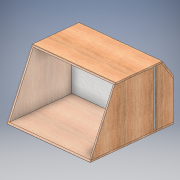
# Autodesk Inventor part: spraybooth
Saved by Autodesk Inventor 2017 (Build 210142000, 142)
## iProperties
Created: 2019-04-06
Part Number: spraybooth
Material: Wood (Birch)
Document SubType Name: Modeling
Designer: Brian
Density: 0.55 g/cm^3
Appearance: Birch - Natural Polished
plywood_thickness: 0.500 in
full_depth: 26.000 in
filter_width: 25.000 in
twobyfour_height: 3.500 in
filter_thickness: 1.000 in
acrylic_thickness: 0.250 in
filter_height: 16.000 in
front_angle: 65.00 deg
plenum_depth: 4.250 in
twobyfour_thickness: 1.500 in
d42: 0.500 in
d86: 25.500 in
d87: 0.00 deg
d90: 1.000 in
d93: 0.500 in
d96: 0.500 in
d102: 0.500 in
d104: 1.000 in
d105: 3.500 in
d106: 1.000 in
d109: 25.000 in
d110: 0.00 deg
d111: 25.000 in
d112: 0.00 deg
d113: 1.500 in
d114: 0.00 deg
d115: 1.500 in
d116: 0.00 deg
d117: 1.000 in
d118: 0.00 deg
d123: 25.500 in
d124: 0.00 deg
d129: 1.000 in
d130: 0.00 deg
d131: 25.000 in
d132: 0.00 deg
d133: 25.000 in
d134: 0.00 deg
d137: 0.500 in
d138: 0.00 deg
d139: 25.500 in
d140: 0.00 deg
d143: 0.00 deg
d144: 1.500 in
d145: 0.00 deg
d146: 0.500 in
d147: 0.00 deg
d148: 25.500 in
d149: 0.00 deg
d150: 0.500 in
d151: 0.00 deg
d152: 0.500 in
d153: 0.00 deg
d154: 0.500 in
d155: 0.00 deg
d156: 0.500 in
d157: 0.00 deg
d158: 0.500 in
d159: 0.00 deg
d160: 0.500 in
d161: 0.00 deg
d59: 6.070 in
d61: 14.020 in
d62: 11.582 in
d63: 18.641 in
d65: 19.517 in
d66: 35.88 deg
d120: 12.056 in
Author: Brian
Autodesk Inventor part; units mm, degrees
ref_plane "YZ Plane" through (0, 0, 0) normal (1, 0, 0) x (0, 1, 0)
ref_plane "XZ Plane" through (0, 0, 0) normal (0, 1, 0) x (-1, 0, 0)
ref_plane "XY Plane" through (0, 0, 0) normal (0, 0, 1) x (1, 0, 0)
sketch "Sketch2" plane through (0, 0, 0) normal (1, 0, 0) x (0, 0, 1)
  line L0 (-641.7779, 0) -> (-641.7779, -290.0603)
  line L1 (-654.4779, -294.1723) -> (-654.4779, 0)
  line L2 (-551.5263, -419.1) -> (-195.4295, -419.1)
  line L3 (5.9221, 12.7) -> (-654.4779, 12.7)
  line L4 (-654.4779, 12.7) -> (-654.4779, 0)
  line L5 (11.6772, 10.0164) -> (5.9221, 12.7)
  line L6 (0, 0) -> (5.9221, 12.7)
  line L7 (-573.2932, -406.4) -> (-654.4779, -294.1723)
  line L8 (-521.1279, -406.4) -> (-533.8279, -406.4)
  line L9 (-533.8279, 0) -> (-521.1279, 0)
  line L10 (-559.2279, -317.5) -> (-533.8279, -317.5)
  line L11 (-533.8279, 0) -> (-559.2279, 0)
  line L12 (-641.7779, -88.9) -> (-533.8279, -88.9)
  line L13 (-521.1279, -406.4) -> (-533.8279, -406.4)
  line L14 (-533.8279, -406.4) -> (-533.8279, -381)
  line L15 (-521.1279, -381) -> (-521.1279, -406.4)
  line L16 (-521.1279, 0) -> (-533.8279, 0)
  line L17 (-533.8279, 0) -> (-533.8279, -25.4)
  line L18 (-533.8279, -25.4) -> (-521.1279, -25.4)
  line L19 (-521.1279, -25.4) -> (-521.1279, 0)
  line L20 (-495.7279, 0) -> (-521.1279, 0)
  line L21 (-551.5263, -419.1) -> (-564.1061, -419.1)
  line L22 (5.9221, 12.7) -> (11.6772, 10.0164)
  line L23 (11.6772, 10.0164) -> (-188.4231, -419.1)
  line L24 (-188.4231, -419.1) -> (-194.1781, -416.4164)
  line L25 (-654.4779, 0) -> (-641.7779, 0)
  line L26 (-641.7779, 0) -> (-654.4779, 0)
  line L27 (-641.7779, 0) -> (-654.4779, 0)
  line L28 (-521.1279, -25.4) -> (-533.8279, -25.4)
  line L29 (-533.8279, 0) -> (-521.1279, 0)
  line L30 (-521.1279, -406.4) -> (-533.8279, -406.4)
  line L31 (-559.2279, -317.5) -> (-533.8279, -317.5)
  line L32 (-533.8279, -88.9) -> (-641.7779, -88.9)
  line L33 (-521.1279, -381) -> (-521.1279, -25.4)
  line L34 (5.9221, 12.7) -> (11.6772, 10.0164)
  line L35 (-521.1279, -406.4) -> (-533.8279, -406.4)
  line L36 (-533.8279, -406.4) -> (-533.8279, -381)
  line L37 (-521.1279, -381) -> (-521.1279, -406.4)
  line L38 (-533.8279, -25.4) -> (-521.1279, -25.4)
  line L39 (-521.1279, -25.4) -> (-521.1279, -381)
  line L40 (-521.1279, -25.4) -> (-533.8279, -25.4)
  line L41 (-533.8279, -25.4) -> (-533.8279, 0)
  line L42 (-533.8279, 0) -> (-521.1279, 0)
  line L43 (-521.1279, 0) -> (-521.1279, -25.4)
  line L44 (-654.4779, -294.1723) -> (-573.2932, -406.4)
  line L45 (-564.1061, -419.1) -> (-551.5263, -419.1)
  line L46 (-533.8279, -406.4) -> (-557.6186, -406.4)
  line L47 (-495.7279, -406.4) -> (-521.1279, -406.4)
  line L48 (-194.1781, -416.4164) -> (0, 0)
  line L49 (-521.1279, -381) -> (-533.8279, -381)
  line L50 (-557.6186, -406.4) -> (-573.2932, -406.4)
  line L51 (-521.1279, -406.4) -> (-495.7279, -406.4)
  line L52 (-495.7279, -406.4) -> (-495.7279, 0)
  line L53 (-189.5074, -406.4) -> (-495.7279, -406.4)
  line L54 (0, 0) -> (-495.7279, 0)
  line L55 (-559.2279, 0) -> (-641.7779, 0)
  line L56 (-533.8279, -25.4) -> (-533.8279, -88.9)
  line L57 (-533.8279, -88.9) -> (-533.8279, -317.5)
  line L58 (-533.8279, -381) -> (-533.8279, -317.5)
  line L59 (-559.2279, -317.5) -> (-621.9282, -317.5)
  line L60 (-557.6186, -406.4) -> (-621.9282, -317.5)
  line L61 (-573.2932, -406.4) -> (-564.1061, -419.1)
  line L62 (-621.9282, -317.5) -> (-654.4779, -272.5041)
  line L63 (-189.5074, -406.4) -> (-189.5074, -406.4)
  line L64 (-189.5074, -406.4) -> (-194.1781, -416.4164)
  line L65 (-195.4295, -419.1) -> (-189.5074, -406.4)
  point P0 (-641.7779, -285.2823)
  dimension "d42" = 12.7
  dimension "full_depth" = 660.4
  dimension "d59" = 154.1882
  dimension "d61" = 356.0967
  dimension "d62" = 294.1723
  dimension "d63" = 473.4775
  dimension "d65" = 495.7279
  dimension "d66" = 35.882
  dimension "d90" = 25.4
  dimension "twobyfour_height" = 88.9
  dimension "d93" = 12.7
  dimension "filter_thickness" = 25.4
  dimension "d96" = 12.7
  dimension "acrylic_thickness" = 6.35
  dimension "d102" = 12.7
  dimension "filter_height" = 406.4
  dimension "d104" = 25.4
  dimension "d105" = 88.9
  dimension "d106" = 25.4
  dimension "front_angle" = 65
  dimension "d120" = 306.2205
  dimension "plenum_depth" = 107.95
  constraints: 135 end point, 15 collinear, 14 horizontal, 13 parallel, 11 perpendicular, 6 point on line, 1 vertical
  measures "d42" distance between parallel lines of L1 L0
  measures "full_depth" distance of L3.start L4.start
  measures "d59" distance of L21.end L1.start
  measures "d61" distance of L2.end L2.start
  measures "d62" distance of L1.end L1.start
  measures "d63" distance of L23.end L5.start
  measures "d65" distance of L6.start L20.start
  measures "d66" angle of L1 L7
  measures "d90" distance between parallel lines of L49 L8
  measures "twobyfour_height" distance between parallel lines of L10 L46
  measures "d93" distance between parallel lines of L2 L53
  measures "filter_thickness" distance between parallel lines of L33 L52
  measures "d96" distance between parallel lines of L14 L37
  measures "acrylic_thickness" distance between parallel lines of L48 L23
  measures "d102" distance between parallel lines of L54 L3
  measures "filter_height" distance between parallel lines of L54 L53
  measures "d104" distance between parallel lines of L16 L28
  measures "d105" distance between parallel lines of L11 L32
  measures "d106" distance of L20.start L9.end
  measures "front_angle" angle of L48 L54
  measures "d120" distance of L53.start L47.start
  measures "plenum_depth" distance between parallel lines of L0 L57
extrude "Extrusion9" add sketch "Sketch2" along normal blind 647.7 contours L5 L23 L24 L48 L6
extrude "Extrusion10" add sketch "Sketch2" along normal blind 635 separate body contours L49 L15 L8 L14
extrude "Extrusion11" add sketch "Sketch2" along normal blind 635 separate body contours L9 L19 L18 L17
extrude "Extrusion12" add sketch "Sketch2" along normal blind 38.1 separate body contours L59 L10 L58 L14 L46 L60
extrude "Extrusion13" add sketch "Sketch2" along normal blind 38.1 separate body contours L55 L11 L17 L56 L12 L0
extrude "Extrusion14" add sketch "Sketch2" along normal blind 25.4 separate body contours L56 L18 L33 L49 L58 L57
extrude "Extrusion15" add sketch "Sketch2" along normal blind 647.7 separate body contours L46 L8 L47 L53 L48 L65 L2 L21 L61 L50
ref_plane "Work Plane3" through (635, 0, 0) normal (1, 0, 0) x (0, 0, -1)
sketch "Sketch5" plane through (635, 0, 0) normal (1, 0, 0) x (0, 0, -1)
  line L0 (533.8279, 88.9) -> (533.8279, 0) projected
  line L1 (533.8279, 0) -> (641.7779, 0) projected
  line L2 (641.7779, 88.9) -> (533.8279, 88.9) projected
  line L3 (557.6186, 406.4) -> (533.8279, 406.4) projected
  line L4 (533.8279, 406.4) -> (533.8279, 317.5) projected
  line L5 (533.8279, 317.5) -> (621.9282, 317.5) projected
  line L6 (533.8279, 0) -> (533.8279, 25.4) projected
  line L7 (533.8279, 25.4) -> (521.1279, 25.4) projected
  line L8 (521.1279, 25.4) -> (521.1279, 0) projected
  line L9 (521.1279, 0) -> (533.8279, 0) projected
  line L10 (521.1279, 406.4) -> (521.1279, 381) projected
  line L11 (521.1279, 381) -> (533.8279, 381) projected
  line L12 (533.8279, 381) -> (533.8279, 406.4) projected
  line L13 (533.8279, 406.4) -> (521.1279, 406.4) projected
  line L14 (533.8279, 25.4) -> (533.8279, 381) projected
  line L15 (533.8279, 381) -> (521.1279, 381) projected
  line L16 (521.1279, 381) -> (521.1279, 25.4) projected
  line L17 (521.1279, 25.4) -> (533.8279, 25.4) projected
  line L18 (641.7779, 88.9) -> (533.8279, 88.9)
  line L19 (533.8279, 88.9) -> (533.8279, 0)
  line L20 (533.8279, 0) -> (559.2279, 0)
  line L21 (533.8279, 381) -> (533.8279, 406.4) projected
  line L22 (533.8279, 355.6) -> (533.8279, 406.4)
  line L23 (533.8279, 406.4) -> (559.2279, 406.4)
  line L24 (521.1279, 406.4) -> (521.1279, 381) projected
  line L25 (521.1279, 406.4) -> (533.8279, 406.4)
  line L26 (533.8279, 406.4) -> (533.8279, 381)
  line L27 (533.8279, 381) -> (521.1279, 381)
  line L28 (521.1279, 381) -> (521.1279, 406.4)
  line L29 (533.8279, 0) -> (533.8279, 25.4) projected
  line L30 (521.1279, 0) -> (533.8279, 0)
  line L31 (533.8279, 0) -> (533.8279, 25.4)
  line L32 (533.8279, 25.4) -> (521.1279, 25.4)
  line L33 (521.1279, 25.4) -> (521.1279, 0)
  line L34 (533.8279, 25.4) -> (521.1279, 25.4) projected
  line L35 (533.8279, 25.4) -> (521.1279, 25.4)
  line L36 (521.1279, 25.4) -> (521.1279, 381)
  line L37 (521.1279, 381) -> (533.8279, 381)
  line L38 (533.8279, 381) -> (533.8279, 25.4)
  line L39 (621.9282, 317.5) -> (557.6186, 406.4) projected
  line L40 (621.9282, 317.5) -> (559.7582, 403.4424)
  line L41 (621.9282, 317.5) -> (533.8279, 317.5)
  line L42 (641.7779, 0) -> (641.7779, 88.9) projected
  line L43 (644.0724, 286.8884) -> (621.9282, 317.5) projected
  line L44 (621.9282, 317.5) -> (654.4779, 272.5041) projected
  line L45 (533.8279, 317.5) -> (621.9282, 317.5) projected
  line L46 (621.9282, 317.5) -> (641.7779, 290.0603)
  line L47 (641.7779, 290.0603) -> (654.4779, 272.5041)
  line L48 (533.8279, 0) -> (641.7779, 0) projected
  line L49 (654.4779, 0) -> (533.8279, 0)
  point P0 (0, 0)
  constraints: 44 end point, 7 parallel, 4 horizontal, 4 perpendicular, 3 collinear, 2 point on line
extrude "Extrusion18" add sketch "Sketch5" against normal blind 25.4 separate body contours L0 L7 L16 L11 L4 L14 | L10 L13 L4 L11
extrude "Extrusion19" add sketch "Sketch2" along normal blind 635 separate body contours L20 L52 L47 L15 L33 L19
extrude "Extrusion20" add sketch "Sketch2" along normal blind 635 separate body contours L0 L62 L1 L25
sketch "Sketch9" plane through (635, 0, 0) normal (1, 0, 0) x (0, 0, -1)
  line L0 (189.5074, 406.4) -> (573.2932, 406.4) projected
  line L1 (564.1061, 419.1) -> (195.4295, 419.1) projected
  line L2 (-11.6772, -10.0164) -> (-5.9221, -12.7) projected
  line L3 (-5.9221, -12.7) -> (194.1781, 416.4164) projected
  line L4 (188.4231, 419.1) -> (-11.6772, -10.0164) projected
  line L5 (654.4779, 0) -> (0, 0) projected
  line L6 (0, 0) -> (-5.9221, -12.7) projected
  line L7 (-5.9221, -12.7) -> (654.4779, -12.7) projected
  line L8 (654.4779, -12.7) -> (654.4779, 0) projected
  line L9 (521.1279, 406.4) -> (495.7279, 406.4) projected
  line L10 (495.7279, 406.4) -> (495.7279, 0) projected
  line L11 (495.7279, 0) -> (521.1279, 0) projected
  line L12 (521.1279, 0) -> (521.1279, 406.4) projected
  line L13 (189.5074, 406.4) -> (495.7279, 406.4)
  line L14 (189.5074, 406.4) -> (573.2932, 406.4) projected
  line L15 (495.7279, 406.4) -> (495.7279, 0) projected
  line L16 (495.7279, 0) -> (0, 0)
  line L17 (189.5074, 406.4) -> (0, 0)
  line L18 (-5.9221, -12.7) -> (194.1781, 416.4164) projected
  line L19 (573.2932, 406.4) -> (564.1061, 419.1) projected
  line L20 (194.1781, 416.4164) -> (188.4231, 419.1) projected
  line L21 (195.4295, 419.1) -> (189.5074, 406.4) projected
  point P0 (560.4163, 406.4)
  point P1 (192.6976, 413.2414)
  point P2 (188.256, 403.7164)
  constraints: 6 end point, 2 collinear, 1 parallel
extrude "Extrusion22" add sketch "Sketch9" along normal blind 12.7 separate body contours L0 L10 L5 L3
extrude "Extrusion23" add sketch "Sketch2" along normal blind 647.7 separate body contours L25 L4 L3 L6 L54 L20 L9 L11 L55
extrude "Extrusion24" add sketch "Sketch5" against normal blind 38.1 separate body contours L2 L42 L1 L0
extrude "Extrusion25" add sketch "Sketch5" against normal blind 38.1 separate body contours L4 L3 L39 L5
sketch "Sketch11" plane through (635, 0, 0) normal (1, 0, 0) x (0, 0, -1)
  line L0 (621.9282, 317.5) -> (654.4779, 272.5041) projected
  line L1 (621.9282, 317.5) -> (557.6186, 406.4) projected
  line L2 (189.5074, 406.4) -> (573.2932, 406.4) projected
  line L3 (533.8279, 381) -> (533.8279, 406.4) projected
  line L4 (533.8279, 406.4) -> (533.8279, 317.5) projected
  line L5 (533.8279, 25.4) -> (533.8279, 406.4) projected
  line L6 (533.8279, 88.9) -> (533.8279, 0) projected
  line L7 (654.4779, 0) -> (0, 0) projected
  line L8 (654.4779, 0) -> (654.4779, 272.5041) projected
  line L9 (521.1279, 25.4) -> (521.1279, 406.4) projected
  line L10 (533.8279, 406.4) -> (557.6186, 406.4) projected
  line L11 (521.1279, 406.4) -> (557.6186, 406.4)
  line L12 (557.6186, 406.4) -> (654.4779, 272.5041)
  line L13 (521.1279, 0) -> (533.8279, 0) projected
  line L14 (654.4779, 0) -> (521.1279, 0)
  line L15 (521.1279, 0) -> (521.1279, 406.4)
  point P0 (189.5074, 406.4)
  constraints: 8 end point, 2 horizontal, 1 perpendicular
extrude "Extrusion26" add sketch "Sketch11" along normal blind 12.7 separate body
extrude "Extrusion27" add sketch "Sketch2" along normal blind 647.7 separate body contours L62 L60 L50 L7 L1
extrude "Extrusion28" add sketch "Sketch2" against normal blind 12.7 contours L46 L8 L47 L53 L48 L65 L2 L21 L61 L50 bodies 7
extrude "Extrusion29" add sketch "Sketch2" against normal blind 12.7 contours L62 L60 L50 L7 L1 bodies 16
extrude "Extrusion30" add sketch "Sketch2" against normal blind 12.7 contours L25 L4 L3 L6 L54 L20 L9 L11 L55 bodies 12
extrude "Extrusion31" add sketch "Sketch2" against normal blind 12.7 contours L5 L23 L24 L48 L6 bodies 1
sketch "Sketch12" plane through (0, 0, 0) normal (-1, 0, 0) x (0, 0, 1)
  line L0 (-195.4295, 419.1) -> (-564.1061, 419.1) projected
  line L1 (-564.1061, 419.1) -> (-573.2932, 406.4) projected
  line L2 (-573.2932, 406.4) -> (-189.5074, 406.4) projected
  line L3 (-573.2932, 406.4) -> (-654.4779, 294.1723) projected
  line L4 (-654.4779, 294.1723) -> (-654.4779, 272.5041) projected
  line L5 (-654.4779, 272.5041) -> (-557.6186, 406.4) projected
  line L6 (-557.6186, 406.4) -> (-573.2932, 406.4) projected
  line L7 (-641.7779, 0) -> (-654.4779, 0) projected
  line L8 (-641.7779, 290.0603) -> (-641.7779, 0) projected
  line L9 (-654.4779, 272.5041) -> (-641.7779, 290.0603) projected
  line L10 (-654.4779, 0) -> (-654.4779, 272.5041) projected
  line L11 (0, 0) -> (-654.4779, 0) projected
  line L12 (-654.4779, 0) -> (-654.4779, -12.7) projected
  line L13 (-654.4779, -12.7) -> (5.9221, -12.7) projected
  line L14 (5.9221, -12.7) -> (0, 0) projected
  line L15 (-557.6186, 406.4) -> (-654.4779, 272.5041)
  line L16 (-654.4779, 0) -> (-654.4779, 272.5041)
  line L17 (-654.4779, 0) -> (0, 0)
  line L18 (0, 0) -> (-189.5074, 406.4)
  line L19 (-557.6186, 406.4) -> (-189.5074, 406.4)
  line L20 (-189.5074, 406.4) -> (-195.4295, 419.1) projected
  constraints: 10 end point, 2 point on line, 1 collinear, 1 parallel, 1 perpendicular
extrude "Extrusion32" add sketch "Sketch12" along normal blind 12.7 separate body contours L18 L11 L8 L5 L2
extrude "Extrusion33" add sketch "Sketch2" against normal blind 12.7 contours L0 L62 L1 L25 bodies 10
body "Solid7"
